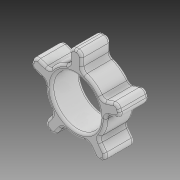
# Autodesk Inventor part: 2102_Tx_Coil_Fins_V1
Saved by Autodesk Inventor 2021 (Build 250183000, 183)
## iProperties
Created: 2022-06-20
Part Number: 2102_Tx_Coil_Fins_V1
Material: Generic
Document SubType Name: Modeling
Designer: Eli
Density: 1 g/cm^3
Appearance: Default
Author: Eli
Autodesk Inventor part; units mm, degrees
ref_plane "YZ Plane" through (0, 0, 0) normal (1, 0, 0) x (0, 1, 0)
ref_plane "XZ Plane" through (0, 0, 0) normal (0, 1, 0) x (-1, 0, 0)
ref_plane "XY Plane" through (0, 0, 0) normal (0, 0, 1) x (1, 0, 0)
sketch "Sketch1" plane through (0, 0, 0) normal (0, 0, 1) x (1, 0, 0)
  circle A0 centre (0, 0) radius 10
  circle A1 centre (0, 0) radius 12.5
  circle A2 centre (0, 0) radius 19 construction
  dimension "d0" = 20
  dimension "d1" = 2.5
  dimension "d2" = 38
  constraints: 3 centre point, 2 coincident
  measures "d0" diameter of A0
  measures "d1" radial gap between concentric circles of A0 A1
  measures "d2" diameter of A2
extrude "Extrusion1" add sketch "Sketch1" along normal blind 12
sketch "Sketch2" plane through (0, 0, 12) normal (0, 0, 1) x (1, 0, 0)
  circle A0 centre (0, 0) radius 12.5 projected
  circle A1 centre (0, 0) radius 12.5 projected
  circle A2 centre (0, 0) radius 19
  line L0 (-2.5, 19) -> (2.5, 19)
  line L1 (2.5, 19) -> (2.5, 0.7124)
  line L2 (2.5, 0.7124) -> (-2.5, 0.7124)
  line L3 (-2.5, 0.7124) -> (-2.5, 19)
  point P0 (0, 19)
  point P1 (-2.5, 18.8348)
  point P2 (-2.5, 12.2474)
  point P3 (2.5, 12.2474)
  point P4 (2.5, 18.8348)
  dimension "d5" = 38
  dimension "d6" = 5
  constraints: 8 end point, 2 parallel, 1 centre point, 1 coincident, 1 horizontal, 1 midpoint, 1 perpendicular, 1 tangent, 1 vertical alignment
  measures "d5" diameter of A2
  measures "d6" distance between parallel lines of L1 L3
extrude "Extrusion2" add sketch "Sketch2" against normal up to surface (12 mm away) contours A0 L3 A2 L1 picked at (0, 14.6479)
fillet "Fillet1" radius 2 4 edges at (2.5, 12.2474, 6) (-2.5, 12.2474, 6) (-2.5, 18.8348, 6) (2.5, 18.8348, 6)
pattern_circular "Circular Pattern1" count 5 over 360 about axis through (0, 0, 0) along (0, 0, 1) of "Extrusion2", "Fillet1"
fillet "Fillet2" radius 1 82 edges at (2.8811, 12.6096, 12) (2.5, 15.3883, 12) (1.9349, 18.3859, 12) (0, 19, 12) (-1.9349, 18.3859, 12) (-2.5, 15.3883, 12) (-2.8811, 12.6096, 12) (-7.3473, 10.1127, 12) (-11.1021, 6.6367, 12) (-13.8626, 7.1329, 12) (-16.8881, 7.5217, 12) (-18.0701, 5.8713, 12) (-18.0839, 3.8414, 12) (-15.4077, 2.3776, 12) (-12.8828, 1.1565, 12) (-11.8882, -3.8627, 12) (-9.7426, -8.5079, 12) (-11.0676, -10.98, 12) (-12.3723, -13.7372, 12) (-11.1679, -15.3713, 12) (-9.2416, -16.0118, 12) (-7.0225, -13.9189, 12) (-5.0808, -11.8949, 12) (0, -12.5, 12) (5.0808, -11.8949, 12) (7.0225, -13.9189, 12) (9.2416, -16.0118, 12) (11.1679, -15.3713, 12) (12.3723, -13.7372, 12) (11.0676, -10.98, 12) (9.7426, -8.5079, 12) (11.8882, -3.8627, 12) (12.8828, 1.1565, 12) (15.4077, 2.3776, 12) (18.0839, 3.8414, 12) (18.0701, 5.8713, 12) (16.8881, 7.5217, 12) (13.8626, 7.1329, 12) (11.1021, 6.6367, 12) (7.3473, 10.1127, 12) (2.8811, 12.6096, 0) (2.5, 15.3883, 0) (1.9349, 18.3859, 0) (0, 19, 0) (-1.9349, 18.3859, 0) (-2.5, 15.3883, 0) (-2.8811, 12.6096, 0) (-7.3473, 10.1127, 0) (-11.1021, 6.6367, 0) (-13.8626, 7.1329, 0) (-16.8881, 7.5217, 0) (-18.0701, 5.8713, 0) (-18.0839, 3.8414, 0) (-15.4077, 2.3776, 0) (-12.8828, 1.1565, 0) (-11.8882, -3.8627, 0) (-9.7426, -8.5079, 0) (-11.0676, -10.98, 0) (-12.3723, -13.7372, 0) (-11.1679, -15.3713, 0) (-9.2416, -16.0118, 0) (-7.0225, -13.9189, 0) (-5.0808, -11.8949, 0) (0, -12.5, 0) (5.0808, -11.8949, 0) (7.0225, -13.9189, 0) (9.2416, -16.0118, 0) (11.1679, -15.3713, 0) (12.3723, -13.7372, 0) (11.0676, -10.98, 0) (9.7426, -8.5079, 0) (11.8882, -3.8627, 0) (12.8828, 1.1565, 0) (15.4077, 2.3776, 0) (18.0839, 3.8414, 0) (18.0701, 5.8713, 0) (16.8881, 7.5217, 0) (13.8626, 7.1329, 0) (11.1021, 6.6367, 0) (7.3473, 10.1127, 0) (-10, 0, 12) (-10, 0, 0)
body "Solid1"
